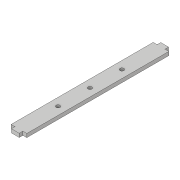
# Autodesk Inventor part: spoonholder
Saved by Autodesk Inventor 2017 (Build 210142000, 142)
## iProperties
Created: 2019-06-11
Part Number: spoonholder
Material: Generic
Document SubType Name: Modeling
Designer: markg
Density: 1 g/cm^3
Appearance: Default
Author: markg
Autodesk Inventor part; units mm, degrees
ref_plane "YZ Plane" through (0, 0, 0) normal (1, 0, 0) x (0, 1, 0)
ref_plane "XZ Plane" through (0, 0, 0) normal (0, 1, 0) x (-1, 0, 0)
ref_plane "XY Plane" through (0, 0, 0) normal (0, 0, 1) x (1, 0, 0)
sketch "Sketch1" plane through (0, 0, 0) normal (0, 1, 0) x (-1, 0, 0)
  line L0 (0, 0) -> (12.7, 0)
  line L1 (12.7, 0) -> (12.7, -115.316)
  line L2 (12.7, -115.316) -> (0, -115.316)
  line L3 (0, -115.316) -> (0, 0)
  line L4 (3.175, 0) -> (9.525, 0)
  line L5 (9.525, 0) -> (9.525, 2.921)
  line L6 (9.525, 2.921) -> (3.175, 2.921)
  line L7 (3.175, 2.921) -> (3.175, 0)
  line L8 (3.175, -115.316) -> (9.525, -115.316)
  line L9 (9.525, -115.316) -> (9.525, -118.237)
  line L10 (9.525, -118.237) -> (3.175, -118.237)
  line L11 (3.175, -118.237) -> (3.175, -115.316)
  dimension "d0" = 115.316
  dimension "d1" = 12.7
  dimension "d2" = 6.35
  dimension "d3" = 3.175
  dimension "d4" = 2.921
  dimension "d5" = 2.921
  dimension "d6" = 3.175
  constraints: 24 end point, 6 parallel, 3 horizontal, 3 perpendicular, 3 point on line
  measures "d0" distance of L0.end L1.end
  measures "d1" distance of L1.end L2.end
  measures "d2" distance of L5.end L6.end
  measures "d3" distance between parallel lines of L3 L7
  measures "d4" distance of L4.end L5.end
  measures "d5" distance of L8.end L9.end
  measures "d6" distance between parallel lines of L3 L11
extrude "Extrusion1" add sketch "Sketch1" along normal blind 2.921
sketch "Sketch2" plane through (0, 2.921, 0) normal (0, 1, 0) x (1, 0, 0)
  circle A0 centre (-6.35, 31.75) radius 1.5875
  circle A1 centre (-6.35, 83.566) radius 1.5875
  line L0 (0, 0) -> (0, 115.316) projected
  line L1 (-3.175, 0) -> (0, 0) projected
  line L2 (0, 115.316) -> (-3.175, 115.316) projected
  dimension "d9" = 3.175
  dimension "d10" = 3.175
  dimension "d11" = 6.35
  dimension "d12" = 6.35
  dimension "d13" = 31.75
  dimension "d14" = 31.75
  constraints: 2 centre point
  measures "d9" diameter of A0
  measures "d10" diameter of A1
  measures "d11" distance from line of L0 A1.centre
  measures "d12" distance from line of L0 A0.centre
  measures "d13" distance from line of A0.centre L1
  measures "d14" distance from line of L2 A1.centre
extrude "Extrusion2" cut sketch "Sketch2" against normal blind 2.921
sketch "Sketch3" plane through (0, 2.921, 0) normal (0, 1, 0) x (1, 0, 0)
  circle A0 centre (-6.35, 57.658) radius 1.5875
  line L0 (0, 0) -> (0, 115.316) projected
  line L1 (-3.175, 0) -> (0, 0) projected
  dimension "d17" = 3.175
  dimension "d18" = 6.35
  dimension "d19" = 57.658
  constraints: 1 centre point
  measures "d17" diameter of A0
  measures "d18" distance from line of L0 A0.centre
  measures "d19" distance from line of L1 A0.centre
extrude "Extrusion3" cut sketch "Sketch3" against normal blind 2.921
body "Solid1"
